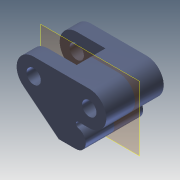
# Autodesk Inventor part: TU-008
Saved by Autodesk Inventor 2011 (Build 150229000, 229)
## iProperties
Shininess: 64.0
Angle Display Precision: 2
Document Length Units: 11269
Document Angle Units: 11279
Document Time Units: 11290
Document Mass Units: 11286
Document Length Units Precision: 3
Document Angle Units Precision: 2
Created: 2002-07-24
Part Number: TU-008
Document SubType Name: Modeling
Designer: PN
Density: 1 g/cm^3
Description: Hinge
Mass: 25.6282 g
Surface Area: 85.6046 cm^2
Volume: 25.6282 cm^3
Density: 0.0
Volumn: 0.0
Area: 0.0
PropertySet Name: Model Information
Control State: 0
Master: False
Checked Out: False
LENGTH: 1.000 in
Author: PN
Autodesk Inventor part; units mm, degrees
ref_plane "YZ Plane" through (0, 0, 0) normal (1, 0, 0) x (0, 1, 0)
ref_plane "XZ Plane" through (0, 0, 0) normal (0, 1, 0) x (-1, 0, 0)
sketch "Sketch1" plane through (0, 0, 0) normal (0, 0, 1) x (1, 0, 0)
  circle A0 centre (31, -9.5) radius 4 construction
  circle A1 centre (0, -9.5) radius 4 construction
  line L0 (31, 0) -> (0, 0)
  arc A2 (0, 0) -> (-5.5818, -17.1873) centre (0, -9.5) ccw
  line L1 (14, -32.8402) -> (-5.5818, -17.1873)
  line L2 (23.513, -32.8402) -> (14, -32.8402)
  arc A3 (23.513, -32.8402) -> (24.6813, -21.9658) centre (23.513, -27.3402) ccw
  arc A4 (25, -19) -> (24.6813, -21.9658) centre (25, -20.5) ccw
  line L3 (31, -19) -> (25, -19)
  arc A5 (31, -19) -> (31, 0) centre (31, -9.5) ccw
  point P0 (0, 0)
  dimension "d0" = 9.5
  dimension "d1" = 8
  dimension "d2" = 31
  dimension "d3" = 1.5
  dimension "d4" = 5.5
  dimension "d6" = 9.513
  dimension "d7" = 38.638
  dimension "d9" = 32.8402
  dimension "d10" = 16.9104
  constraints: 8 end point, 8 point on circle, 7 tangent, 6 centre point, 2 coincident with centre, 2 parallel, 1 coincident, 1 equal radius, 1 horizontal
  measures "d0" radius of A2
  measures "d1" diameter of A1
  measures "d2" distance of A5.centre A2.centre
  measures "d3" radius of A4
  measures "d4" radius of A3
  measures "d6" distance of L2.start L1.start
  measures "d7" angle of L2 L1
  measures "d9" distance between parallel lines of L2 L0
  measures "d10" distance from line of point (0, 0) L1
extrude "Extrusion1" add sketch "Sketch1" along normal mid plane 32
sketch "Sketch2" plane through (14, -32.8402, 16) normal (0, -1, 0) x (1, 0, 0)
  line L0 (0, -32) -> (0, 0) projected
  line L1 (-23.5, -32) -> (-23.5, 0) projected
  line L2 (-23.5, -24) -> (2, -24)
  line L3 (2, -24) -> (2, -8)
  line L4 (2, -8) -> (-23.5, -8)
  line L5 (-23.5, -8) -> (-23.5, -24)
  point P0 (-23.5, -16)
  dimension "d13" = 2
  dimension "d14" = 16
  constraints: 8 end point, 2 midpoint, 2 parallel, 1 horizontal, 1 perpendicular
  measures "d13" distance between parallel lines of L3 L0
  measures "d14" distance of L4.end L2.start
extrude "Extrusion2" cut sketch "Sketch2" against normal through all
hole "Hole1" at (31, -9.5, 16) direction (0, 0, -1) diameter 8 end through all
hole "Hole2" at (0, -9.5, 16) direction (0, 0, -1) diameter 8 end through all
equation "\"LENGTH\" = 25.4"
body "Solid1"
